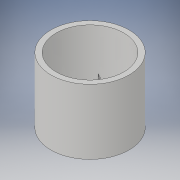
# Autodesk Inventor part: Whistle Splitter 30mmR
Saved by Autodesk Inventor 2019 (Build 230136000, 136)
## iProperties
Created: 2020-04-08
Part Number: Whistle Splitter 30mmR
Material: Generic
Document SubType Name: Modeling
Designer: Kepler
Density: 1 g/cm^3
Appearance: Default
Author: Kepler
Autodesk Inventor part; units mm, degrees
ref_plane "YZ Plane" through (0, 0, 0) normal (1, 0, 0) x (0, 1, 0)
ref_plane "XZ Plane" through (0, 0, 0) normal (0, 1, 0) x (-1, 0, 0)
ref_plane "XY Plane" through (0, 0, 0) normal (0, 0, 1) x (1, 0, 0)
sketch "Sketch1" plane through (0, 0, 0) normal (0, 1, 0) x (-1, 0, 0)
  circle A0 centre (0, 0) radius 30
  circle A1 centre (0, 0) radius 26
  dimension "d0" = 60
  dimension "d1" = 52
  constraints: 2 centre point, 2 coincident
  measures "d0" diameter of A0
  measures "d1" diameter of A1
extrude "Extrusion1" add sketch "Sketch1" along normal blind 50
sketch "Sketch2" plane through (0, 0, 0) normal (1, 0, 0) x (0, 1, 0)
  line L0 (0, 30) -> (0, -30) projected
  line L1 (0, -26) -> (19.3804, -20.807)
  line L2 (0, -26) -> (20.8201, -31.5787)
  line L3 (19.3804, -20.807) -> (-2.465, -20.807)
  line L4 (-2.465, -20.807) -> (-2.465, -32.37)
  line L5 (-2.465, -32.37) -> (20.8201, -32.37)
  line L6 (20.8201, -32.37) -> (20.8201, -31.5787)
  line L7 (0, -26) -> (50, -26) projected
  point P0 (0, 0)
  dimension "d6" = 15
  dimension "d7" = 15
  constraints: 12 end point, 3 perpendicular, 1 horizontal
  measures "d6" angle of L2 L7
  measures "d7" angle of L7 L1
extrude "Extrusion2" cut sketch "Sketch2" along normal mid plane 30
body "Solid1"
